Trimix_Enclosure_A3_PrintReview (Autodesk Fusion 360 design; units mm, degrees)
description: Main housing
part number: TMX-A3-P01
description: Single rear cover
part number: TMX-A3-P02
description: Guition display assembly
part number: TMX-A3-C01-V01
part number: TMX-A3-C01-V02
part number: TMX-A3-C01-V03
part number: TMX-A3-C01-V04
description: M3 x 8 button-head screw
part number: TMX-A3-F01
description: M3 heat-set insert, OD4.2 x 5
part number: TMX-A3-F04
description: Electronics carrier
part number: TMX-A3-P03
description: Main electronics PCB
part number: TMX-A3-B01
description: M2 x 7 socket-cap screw
part number: TMX-A3-F03
description: M2 heat-set insert, OD3.2 x 4
part number: TMX-A3-F05
description: Lower display retainer
part number: TMX-A3-P04
description: Upper display retainer
part number: TMX-A3-P05
description: M2 x 5 socket-cap screw
part number: TMX-A3-F02
description: Protected two-cell holder
part number: TMX-A3-C02
description: 18650 cell
part number: TMX-A3-C03-V01
part number: TMX-A3-C03-V02
description: Two-wire battery disconnect pair
part number: TMX-A3-C10-V01
part number: TMX-A3-C10-V02
description: Momentary illuminated 1NO button
part number: TMX-A3-C04-V01
part number: TMX-A3-C04-V02
part number: TMX-A3-C04-V03
description: Printed USB bezel and hidden flange
part number: TMX-A3-P09
description: USB support frame
part number: TMX-A3-P06
description: Printed USB retaining bridge
part number: TMX-A3-P10
description: USB daughterboard
part number: TMX-A3-B02
description: USB-C receptacle
part number: TMX-A3-C05-V01
part number: TMX-A3-C05-V02
part number: TMX-A3-C05-V04
part number: TMX-A3-C05-V03
description: Sampling manifold
part number: TMX-A3-P07
description: Sampling chamber lid
part number: TMX-A3-P08
description: AO2 threaded adapter
part number: TMX-A3-P11
description: Oxygen sensor
part number: TMX-A3-C06
description: AO2 mating cable/connector
part number: TMX-A3-C12
description: Carbon-monoxide module
part number: TMX-A3-C09
description: Thermal-conductivity sensor
part number: TMX-A3-C07
description: Humidity breakout
part number: TMX-A3-C08
description: Gas fitting
part number: TMX-A3-C11-V01
part number: TMX-A3-C11-V02
description: AO2 face seal
part number: TMX-A3-S02
description: Chamber harness closure
part number: TMX-A3-S01
description: Guition 4.3 inch display assembly
part number: TMX-A3-C01
description: Momentary 1NO button assembly
part number: TMX-A3-C04
description: GCT USB4720-03-A connector assembly
part number: TMX-A3-C05
Autodesk Fusion 360 part; units mm, degrees
(part 1 of 7)
ref_plane "WorkPlane1" through (0, 0, 0) normal (0, 0, 1) x (1, 0, 0) in component "01 Shape A housing"
sketch "Flat front Shape A outline" plane through (0, 0, 0) normal (0, 0, 1) x (1, 0, 0) in component "01 Shape A housing"
  line L0 (0, 0) -> (85, 0)
  line L1 (85, 0) -> (85, 180)
  line L2 (85, 180) -> (0, 180)
  line L3 (0, 180) -> (0, 0)
  dimension "d39" = 85
  dimension "d40" = 180
  constraint horizontal L0
  constraint vertical L1
  constraint horizontal L2
  constraint vertical L3
  measures "d39" horizontal distance of L0.start L0.end
  measures "d40" vertical distance of L0.end L1.end
ref_plane "WorkPlane2" through (0, 0, 40.6) normal (0, 0, 1) x (1, 0, 0) in component "01 Shape A housing"
sketch "Gently tapered rear outline" plane through (0, 0, 40.6) normal (0, 0, 1) x (1, 0, 0) in component "01 Shape A housing"
  line L0 (0.25, 0.25) -> (84.75, 0.25)
  line L1 (84.75, 0.25) -> (84.75, 179.75)
  line L2 (84.75, 179.75) -> (0.25, 179.75)
  line L3 (0.25, 179.75) -> (0.25, 0.25)
  dimension "d43" = 0.25
  dimension "d44" = 0.25
  dimension "d45" = 84.5
  dimension "d46" = 179.5
  constraint horizontal L0
  constraint vertical L1
  constraint horizontal L2
  constraint vertical L3
  measures "d43" horizontal distance of origin L0.start
  measures "d44" vertical distance of origin L0.start
  measures "d45" horizontal distance of L0.start L0.end
  measures "d46" vertical distance of L0.end L1.end
loft "Shape A restrained taper" add profiles "Flat front Shape A outline", "Gently tapered rear outline" section 1 contours L0 L1 L2 L3 picked at (28.333333, 120) section 2 contours L0 L1 L2 L3 picked at (28.416667, 60.083333) makes body 1 in component "01 Shape A housing"
fillet "Shape A soft outer corners" radius 8 4 edges at (0.125, 0.125, 20.3) (0.125, 179.875, 20.3) (84.875, 0.125, 20.3) (84.875, 179.875, 20.3) on bodies 1 in component "01 Shape A housing"
ref_plane "WorkPlane3" through (0, 0, 14.5) normal (0, 0, 1) x (1, 0, 0) in component "01 Shape A housing"
sketch "Rear cavity cutting tool sketch" plane through (0, 0, 14.5) normal (0, 0, 1) x (1, 0, 0) in component "01 Shape A housing"
  line L0 (2.4, 2.4) -> (82.6, 2.4)
  line L1 (82.6, 2.4) -> (82.6, 177.6)
  line L2 (82.6, 177.6) -> (2.4, 177.6)
  line L3 (2.4, 177.6) -> (2.4, 2.4)
  dimension "d51" = 2.4
  dimension "d52" = 2.4
  dimension "d53" = 80.2
  dimension "d54" = 175.2
  constraint horizontal L0
  constraint vertical L1
  constraint horizontal L2
  constraint vertical L3
  measures "d51" horizontal distance of origin L0.start
  measures "d52" vertical distance of origin L0.start
  measures "d53" horizontal distance of L0.start L0.end
  measures "d54" vertical distance of L0.end L1.end
extrude "Rear cavity cutting tool" add sketch "Rear cavity cutting tool sketch" along normal blind 43 separate body contours L0 L1 L2 L3 picked at (29.133333, 60.8) makes body 2 in component "01 Shape A housing"
fillet "Inner cavity corner rounds" radius 5.6 4 edges at (2.4, 177.6, 36) (82.6, 177.6, 36) (82.6, 2.4, 36) (2.4, 2.4, 36) on bodies 2 in component "01 Shape A housing"
combine "Rounded rear electronics cavity" operation cut target body 1 tool bodies 2 in component "01 Shape A housing"
ref_plane "WorkPlane4" through (0, 0, 2.4) normal (0, 0, 1) x (1, 0, 0) in component "01 Shape A housing"
sketch "Upper sensor cavity cutting tool sketch" plane through (0, 0, 2.4) normal (0, 0, 1) x (1, 0, 0) in component "01 Shape A housing"
  line L0 (2.4, 128) -> (82.6, 128)
  line L1 (82.6, 128) -> (82.6, 177.6)
  line L2 (82.6, 177.6) -> (2.4, 177.6)
  line L3 (2.4, 177.6) -> (2.4, 128)
  dimension "d61" = 2.4
  dimension "d62" = 128
  dimension "d63" = 80.2
  dimension "d64" = 49.6
  constraint horizontal L0
  constraint vertical L1
  constraint horizontal L2
  constraint vertical L3
  measures "d61" horizontal distance of origin L0.start
  measures "d62" vertical distance of origin L0.start
  measures "d63" horizontal distance of L0.start L0.end
  measures "d64" vertical distance of L0.end L1.end
extrude "Upper sensor cavity cutting tool" add sketch "Upper sensor cavity cutting tool sketch" along normal blind 43 separate body contours L0 L1 L2 L3 picked at (29.133333, 161.066667) makes body 3 in component "01 Shape A housing"
fillet "Upper pod inner top corner rounds" radius 5.6 2 edges at (2.4, 177.6, 23.9) (82.6, 177.6, 23.9) on bodies 3 in component "01 Shape A housing"
combine "Upper sensor pod front clearance" operation cut target body 1 tool bodies 3 in component "01 Shape A housing"
ref_plane "WorkPlane5" through (0, 0, -1) normal (0, 0, 1) x (1, 0, 0) in component "01 Shape A housing"
sketch "Front removable factory display aperture sketch" plane through (0, 0, -1) normal (0, 0, 1) x (1, 0, 0) in component "01 Shape A housing"
  line L0 (7.45, 4.8) -> (77.55, 4.8)
  line L1 (77.55, 4.8) -> (77.55, 122.4)
  line L2 (77.55, 122.4) -> (7.45, 122.4)
  line L3 (7.45, 122.4) -> (7.45, 4.8)
  dimension "d71" = 7.45
  dimension "d72" = 4.8
  dimension "d73" = 70.1
  dimension "d74" = 117.6
  constraint horizontal L0
  constraint vertical L1
  constraint horizontal L2
  constraint vertical L3
  measures "d71" horizontal distance of origin L0.start
  measures "d72" vertical distance of origin L0.start
  measures "d73" horizontal distance of L0.start L0.end
  measures "d74" vertical distance of L0.end L1.end
extrude "Front removable factory display aperture" cut sketch "Front removable factory display aperture sketch" along normal blind 16 contours L0 L1 L2 L3 picked at (30.816667, 83.2) bodies 1 in component "01 Shape A housing"
fillet "Display aperture corner rounds" radius 2.4 4 edges at (77.55, 4.8, 7.25) (7.45, 4.8, 7.25) (7.45, 122.4, 7.25) (77.55, 122.4, 7.25) on bodies 1 in component "01 Shape A housing"
ref_plane "WorkPlane6" through (-1, 0, 0) normal (1, 0, 0) x (0, 1, 0) in component "01 Shape A housing"
sketch "Opposed upper gas fitting clearances sketch" plane through (-1, 0, 0) normal (1, 0, 0) x (0, 0, -1) in component "01 Shape A housing"
  circle A0 centre (-22, 162.5) radius 4.5
  dimension "d82" = 162.5
  dimension "d83" = 4.5
  measures "d82" vertical distance of origin A0.centre
  measures "d83" radius of A0
extrude "Opposed upper gas fitting clearances" cut sketch "Opposed upper gas fitting clearances sketch" along normal blind 87 contours A0 picked at (-22.333781, 163.962392) bodies 1 in component "01 Shape A housing"
ref_plane "WorkPlane7" through (81.6, 0, 0) normal (1, 0, 0) x (0, 1, 0) in component "01 Shape A housing"
sketch "Left-side power button opening sketch" plane through (81.6, 0, 0) normal (1, 0, 0) x (0, 0, -1) in component "01 Shape A housing"
  circle A0 centre (-31, 113) radius 6
  dimension "d89" = 113
  dimension "d90" = 6
  measures "d89" vertical distance of origin A0.centre
  measures "d90" radius of A0
extrude "Left-side power button opening" cut sketch "Left-side power button opening sketch" along normal blind 4.4 contours A0 picked at (-29.46738, 110.75206) bodies 1 in component "01 Shape A housing"
ref_plane "WorkPlane1" through (0, 0, 40.8) normal (0, 0, 1) x (1, 0, 0) in component "02 Single rear cover"
sketch "Single rear cover sketch" plane through (0, 0, 40.8) normal (0, 0, 1) x (1, 0, 0) in component "02 Single rear cover"
  line L0 (0.25, 0.25) -> (84.75, 0.25)
  line L1 (84.75, 0.25) -> (84.75, 179.75)
  line L2 (84.75, 179.75) -> (0.25, 179.75)
  line L3 (0.25, 179.75) -> (0.25, 0.25)
  dimension "d95" = 0.25
  dimension "d96" = 0.25
  dimension "d97" = 84.5
  dimension "d98" = 179.5
  constraint horizontal L0
  constraint vertical L1
  constraint horizontal L2
  constraint vertical L3
  measures "d95" horizontal distance of origin L0.start
  measures "d96" vertical distance of origin L0.start
  measures "d97" horizontal distance of L0.start L0.end
  measures "d98" vertical distance of L0.end L1.end
extrude "Single rear cover" add sketch "Single rear cover sketch" along normal blind 2.2 separate body contours L0 L1 L2 L3 picked at (28.416667, 60.083333) makes body 4 in component "02 Single rear cover"
fillet "Soft rear cover corners" radius 8 4 edges at (0.25, 179.75, 41.9) (84.75, 179.75, 41.9) (84.75, 0.25, 41.9) (0.25, 0.25, 41.9) on bodies 4 in component "02 Single rear cover"
fillet "Soft rear edge roll" radius 0.8 8 edges at (2.593146, 2.593146, 43) (0.25, 90, 43) (42.5, 0.25, 43) (82.406854, 2.593146, 43) (84.75, 90, 43) (82.406854, 177.406854, 43) (42.5, 179.75, 43) (2.593146, 177.406854, 43) on bodies 4 in component "02 Single rear cover"
ref_plane "WorkPlane1" through (0, 0, 0.4) normal (0, 0, 1) x (1, 0, 0) in component "03 Guition factory casing — measured envelope"
sketch "Retained factory frame sketch" plane through (0, 0, 0.4) normal (0, 0, 1) x (1, 0, 0) in component "03 Guition factory casing — measured envelope"
  line L0 (7.85, 5.2) -> (77.15, 5.2)
  line L1 (77.15, 5.2) -> (77.15, 122)
  line L2 (77.15, 122) -> (7.85, 122)
  line L3 (7.85, 122) -> (7.85, 5.2)
  dimension "d107" = 7.85
  dimension "d108" = 5.2
  dimension "d109" = 69.3
  dimension "d110" = 116.8
  constraint horizontal L0
  constraint vertical L1
  constraint horizontal L2
  constraint vertical L3
  measures "d107" horizontal distance of origin L0.start
  measures "d108" vertical distance of origin L0.start
  measures "d109" horizontal distance of L0.start L0.end
  measures "d110" vertical distance of L0.end L1.end
extrude "Retained factory frame" add sketch "Retained factory frame sketch" along normal blind 13.7 separate body contours L0 L1 L2 L3 picked at (30.95, 83.066667) makes body 5 in component "03 Guition factory casing — measured envelope"
fillet "Factory corner reference" radius 2 4 edges at (7.85, 122, 7.25) (77.15, 122, 7.25) (77.15, 5.2, 7.25) (7.85, 5.2, 7.25) on bodies 5 in component "03 Guition factory casing — measured envelope"
ref_plane "WorkPlane2" through (0, 0, 3.4) normal (0, 0, 1) x (1, 0, 0) in component "03 Guition factory casing — measured envelope"
sketch "Factory open rear sketch" plane through (0, 0, 3.4) normal (0, 0, 1) x (1, 0, 0) in component "03 Guition factory casing — measured envelope"
  line L0 (9.8, 9.6) -> (75.2, 9.6)
  line L1 (75.2, 9.6) -> (75.2, 117.6)
  line L2 (75.2, 117.6) -> (9.8, 117.6)
  line L3 (9.8, 117.6) -> (9.8, 9.6)
  dimension "d117" = 9.8
  dimension "d118" = 9.6
  dimension "d119" = 65.4
  dimension "d120" = 108
  constraint horizontal L0
  constraint vertical L1
  constraint horizontal L2
  constraint vertical L3
  measures "d117" horizontal distance of origin L0.start
  measures "d118" vertical distance of origin L0.start
  measures "d119" horizontal distance of L0.start L0.end
  measures "d120" vertical distance of L0.end L1.end
extrude "Factory open rear" cut sketch "Factory open rear sketch" along normal blind 12 contours L0 L1 L2 L3 picked at (31.6, 81.6) bodies 5 in component "03 Guition factory casing — measured envelope"
ref_plane "WorkPlane3" through (0, 0, 0.3) normal (0, 0, 1) x (1, 0, 0) in component "03 Guition factory casing — measured envelope"
sketch "Factory glass recess sketch" plane through (0, 0, 0.3) normal (0, 0, 1) x (1, 0, 0) in component "03 Guition factory casing — measured envelope"
  line L0 (9.1, 6.4) -> (75.9, 6.4)
  line L1 (75.9, 6.4) -> (75.9, 120.8)
  line L2 (75.9, 120.8) -> (9.1, 120.8)
  line L3 (9.1, 120.8) -> (9.1, 6.4)
  dimension "d125" = 9.1
  dimension "d126" = 6.4
  dimension "d127" = 66.8
  dimension "d128" = 114.4
  constraint horizontal L0
  constraint vertical L1
  constraint horizontal L2
  constraint vertical L3
  measures "d125" horizontal distance of origin L0.start
  measures "d126" vertical distance of origin L0.start
  measures "d127" horizontal distance of L0.start L0.end
  measures "d128" vertical distance of L0.end L1.end
extrude "Factory glass recess" cut sketch "Factory glass recess sketch" along normal blind 1.3 contours L0 L1 L2 L3 picked at (31.366667, 82.666667) bodies 5 in component "03 Guition factory casing — measured envelope"
ref_plane "WorkPlane1" through (0, 0, 0.4) normal (0, 0, 1) x (1, 0, 0) in component "04 Guition front glass — drawing reference"
sketch "Factory glass black border sketch" plane through (0, 0, 0.4) normal (0, 0, 1) x (1, 0, 0) in component "04 Guition front glass — drawing reference"
  line L0 (9.1, 6.4) -> (75.9, 6.4)
  line L1 (75.9, 6.4) -> (75.9, 120.8)
  line L2 (75.9, 120.8) -> (9.1, 120.8)
  line L3 (9.1, 120.8) -> (9.1, 6.4)
  dimension "d133" = 9.1
  dimension "d134" = 6.4
  dimension "d135" = 66.8
  dimension "d136" = 114.4
  constraint horizontal L0
  constraint vertical L1
  constraint horizontal L2
  constraint vertical L3
  measures "d133" horizontal distance of origin L0.start
  measures "d134" vertical distance of origin L0.start
  measures "d135" horizontal distance of L0.start L0.end
  measures "d136" vertical distance of L0.end L1.end
extrude "Factory glass black border" add sketch "Factory glass black border sketch" along normal blind 1.2 separate body contours L0 L1 L2 L3 picked at (31.366667, 82.666667) makes body 6 in component "04 Guition front glass — drawing reference"
ref_plane "WorkPlane2" through (0, 0, 0.3) normal (0, 0, 1) x (1, 0, 0) in component "04 Guition front glass — drawing reference"
sketch "Active face recess sketch" plane through (0, 0, 0.3) normal (0, 0, 1) x (1, 0, 0) in component "04 Guition front glass — drawing reference"
  line L0 (14.42, 16.8) -> (70.58, 16.8)
  line L1 (70.58, 16.8) -> (70.58, 110.4)
  line L2 (70.58, 110.4) -> (14.42, 110.4)
  line L3 (14.42, 110.4) -> (14.42, 16.8)
  dimension "d141" = 14.42
  dimension "d142" = 16.8
  dimension "d143" = 56.16
  dimension "d144" = 93.6
  constraint horizontal L0
  constraint vertical L1
  constraint horizontal L2
  constraint vertical L3
  measures "d141" horizontal distance of origin L0.start
  measures "d142" vertical distance of origin L0.start
  measures "d143" horizontal distance of L0.start L0.end
  measures "d144" vertical distance of L0.end L1.end
extrude "Active face recess" cut sketch "Active face recess sketch" along normal blind 0.2 contours L0 L1 L2 L3 picked at (33.14, 48) bodies 6 in component "04 Guition front glass — drawing reference"
ref_plane "WorkPlane1" through (0, 0, 0.4) normal (0, 0, 1) x (1, 0, 0) in component "05 Active 4.3 inch screen"
sketch "Active480x800 screen sketch" plane through (0, 0, 0.4) normal (0, 0, 1) x (1, 0, 0) in component "05 Active 4.3 inch screen"
  line L0 (14.42, 16.8) -> (70.58, 16.8)
  line L1 (70.58, 16.8) -> (70.58, 110.4)
  line L2 (70.58, 110.4) -> (14.42, 110.4)
  line L3 (14.42, 110.4) -> (14.42, 16.8)
  dimension "d149" = 14.42
  dimension "d150" = 16.8
  dimension "d151" = 56.16
  dimension "d152" = 93.6
  constraint horizontal L0
  constraint vertical L1
  constraint horizontal L2
  constraint vertical L3
  measures "d149" horizontal distance of origin L0.start
  measures "d150" vertical distance of origin L0.start
  measures "d151" horizontal distance of L0.start L0.end
  measures "d152" vertical distance of L0.end L1.end
extrude "Active480x800 screen" add sketch "Active480x800 screen sketch" along normal blind 0.1 separate body contours L0 L1 L2 L3 picked at (33.14, 48) makes body 7 in component "05 Active 4.3 inch screen"
ref_plane "WorkPlane1" through (0, 0, 8) normal (0, 0, 1) x (1, 0, 0) in component "06 Guition PCB and connectors — illustrative detail"
sketch "Guition PCB outline sketch" plane through (0, 0, 8) normal (0, 0, 1) x (1, 0, 0) in component "06 Guition PCB and connectors — illustrative detail"
  line L0 (9.97, 9.6) -> (75.03, 9.6)
  line L1 (75.03, 9.6) -> (75.03, 117.6)
  line L2 (75.03, 117.6) -> (9.97, 117.6)
  line L3 (9.97, 117.6) -> (9.97, 9.6)
  dimension "d157" = 9.97
  dimension "d158" = 9.6
  dimension "d159" = 65.06
  dimension "d160" = 108
  constraint horizontal L0
  constraint vertical L1
  constraint horizontal L2
  constraint vertical L3
  measures "d157" horizontal distance of origin L0.start
  measures "d158" vertical distance of origin L0.start
  measures "d159" horizontal distance of L0.start L0.end
  measures "d160" vertical distance of L0.end L1.end
extrude "Guition PCB outline" add sketch "Guition PCB outline sketch" along normal blind 1.6 separate body contours L0 L1 L2 L3 picked at (31.656667, 81.6) makes body 8 in component "06 Guition PCB and connectors — illustrative detail"
ref_plane "WorkPlane2" through (0, 0, 7.9) normal (0, 0, 1) x (1, 0, 0) in component "06 Guition PCB and connectors — illustrative detail"
sketch "Factory mounting-hole reference sketch" plane through (0, 0, 7.9) normal (0, 0, 1) x (1, 0, 0) in component "06 Guition PCB and connectors — illustrative detail"
  circle A0 centre (12.5, 12.3) radius 2.5
  dimension "d165" = 12.5
  dimension "d166" = 12.3
  dimension "d167" = 2.5
  measures "d165" horizontal distance of origin A0.centre
  measures "d166" vertical distance of origin A0.centre
  measures "d167" radius of A0
extrude "Factory mounting-hole reference" cut sketch "Factory mounting-hole reference sketch" along normal blind 1.8 contours A0 picked at (11.518255, 11.733189) bodies 8 in component "06 Guition PCB and connectors — illustrative detail"
ref_plane "WorkPlane3" through (0, 0, 7.9) normal (0, 0, 1) x (1, 0, 0) in component "06 Guition PCB and connectors — illustrative detail"
sketch "Factory mounting-hole reference sketch (1)" plane through (0, 0, 7.9) normal (0, 0, 1) x (1, 0, 0) in component "06 Guition PCB and connectors — illustrative detail"
  circle A0 centre (12.5, 114.9) radius 2.5
  dimension "d172" = 12.5
  dimension "d173" = 114.9
  dimension "d174" = 2.5
  measures "d172" horizontal distance of origin A0.centre
  measures "d173" vertical distance of origin A0.centre
  measures "d174" radius of A0
extrude "Factory mounting-hole reference (1)" cut sketch "Factory mounting-hole reference sketch (1)" along normal blind 1.8 contours A0 picked at (13.287535, 115.621688) bodies 8 in component "06 Guition PCB and connectors — illustrative detail"
ref_plane "WorkPlane4" through (0, 0, 7.9) normal (0, 0, 1) x (1, 0, 0) in component "06 Guition PCB and connectors — illustrative detail"
sketch "Factory mounting-hole reference sketch (2)" plane through (0, 0, 7.9) normal (0, 0, 1) x (1, 0, 0) in component "06 Guition PCB and connectors — illustrative detail"
  circle A0 centre (72.5, 12.3) radius 2.5
  dimension "d179" = 72.5
  dimension "d180" = 12.3
  dimension "d181" = 2.5
  measures "d179" horizontal distance of origin A0.centre
  measures "d180" vertical distance of origin A0.centre
  measures "d181" radius of A0
extrude "Factory mounting-hole reference (2)" cut sketch "Factory mounting-hole reference sketch (2)" along normal blind 1.8 contours A0 picked at (72.060056, 13.42096) bodies 8 in component "06 Guition PCB and connectors — illustrative detail"
ref_plane "WorkPlane5" through (0, 0, 7.9) normal (0, 0, 1) x (1, 0, 0) in component "06 Guition PCB and connectors — illustrative detail"
sketch "Factory mounting-hole reference sketch (3)" plane through (0, 0, 7.9) normal (0, 0, 1) x (1, 0, 0) in component "06 Guition PCB and connectors — illustrative detail"
  circle A0 centre (72.5, 114.9) radius 2.5
  dimension "d186" = 72.5
  dimension "d187" = 114.9
  dimension "d188" = 2.5
  measures "d186" horizontal distance of origin A0.centre
  measures "d187" vertical distance of origin A0.centre
  measures "d188" radius of A0
extrude "Factory mounting-hole reference (3)" cut sketch "Factory mounting-hole reference sketch (3)" along normal blind 1.8 contours A0 picked at (74.260267, 114.705637) bodies 8 in component "06 Guition PCB and connectors — illustrative detail"
ref_plane "WorkPlane6" through (0, 0, 9.6) normal (0, 0, 1) x (1, 0, 0) in component "06 Guition PCB and connectors — illustrative detail"
sketch "ESP32-P4 visual reference sketch" plane through (0, 0, 9.6) normal (0, 0, 1) x (1, 0, 0) in component "06 Guition PCB and connectors — illustrative detail"
  line L0 (20, 76.1) -> (36, 76.1)
  line L1 (36, 76.1) -> (36, 92.1)
  line L2 (36, 92.1) -> (20, 92.1)
  line L3 (20, 92.1) -> (20, 76.1)
  dimension "d193" = 20
  dimension "d194" = 76.1
  dimension "d195" = 16
  dimension "d196" = 16
  constraint horizontal L0
  constraint vertical L1
  constraint horizontal L2
  constraint vertical L3
  measures "d193" horizontal distance of origin L0.start
  measures "d194" vertical distance of origin L0.start
  measures "d195" horizontal distance of L0.start L0.end
  measures "d196" vertical distance of L0.end L1.end
extrude "ESP32-P4 visual reference" add sketch "ESP32-P4 visual reference sketch" along normal blind 3 separate body contours L0 L1 L2 L3 picked at (25.333333, 86.766667) makes body 9 in component "06 Guition PCB and connectors — illustrative detail"
ref_plane "WorkPlane7" through (0, 0, 9.6) normal (0, 0, 1) x (1, 0, 0) in component "06 Guition PCB and connectors — illustrative detail"
sketch "ESP32-C6 visual reference sketch" plane through (0, 0, 9.6) normal (0, 0, 1) x (1, 0, 0) in component "06 Guition PCB and connectors — illustrative detail"
  line L0 (52, 91.1) -> (66, 91.1)
  line L1 (66, 91.1) -> (66, 110.1)
  line L2 (66, 110.1) -> (52, 110.1)
  line L3 (52, 110.1) -> (52, 91.1)
  dimension "d201" = 52
  dimension "d202" = 91.1
  dimension "d203" = 14
  dimension "d204" = 19
  constraint horizontal L0
  constraint vertical L1
  constraint horizontal L2
  constraint vertical L3
  measures "d201" horizontal distance of origin L0.start
  measures "d202" vertical distance of origin L0.start
  measures "d203" horizontal distance of L0.start L0.end
  measures "d204" vertical distance of L0.end L1.end
extrude "ESP32-C6 visual reference" add sketch "ESP32-C6 visual reference sketch" along normal blind 2.8 separate body contours L0 L1 L2 L3 picked at (56.666667, 103.766667) makes body 10 in component "06 Guition PCB and connectors — illustrative detail"
ref_plane "WorkPlane8" through (0, 0, 9.6) normal (0, 0, 1) x (1, 0, 0) in component "06 Guition PCB and connectors — illustrative detail"
sketch "Memory visual reference sketch" plane through (0, 0, 9.6) normal (0, 0, 1) x (1, 0, 0) in component "06 Guition PCB and connectors — illustrative detail"
  line L0 (39, 80.1) -> (46, 80.1)
  line L1 (46, 80.1) -> (46, 89.1)
  line L2 (46, 89.1) -> (39, 89.1)
  line L3 (39, 89.1) -> (39, 80.1)
  dimension "d209" = 39
  dimension "d210" = 80.1
  dimension "d211" = 7
  dimension "d212" = 9
  constraint horizontal L0
  constraint vertical L1
  constraint horizontal L2
  constraint vertical L3
  measures "d209" horizontal distance of origin L0.start
  measures "d210" vertical distance of origin L0.start
  measures "d211" horizontal distance of L0.start L0.end
  measures "d212" vertical distance of L0.end L1.end
extrude "Memory visual reference" add sketch "Memory visual reference sketch" along normal blind 1.2 separate body contours L0 L1 L2 L3 picked at (41.333333, 83.1) makes body 11 in component "06 Guition PCB and connectors — illustrative detail"
ref_plane "WorkPlane9" through (0, 0, 9.6) normal (0, 0, 1) x (1, 0, 0) in component "06 Guition PCB and connectors — illustrative detail"
sketch "Power inductor visual reference sketch" plane through (0, 0, 9.6) normal (0, 0, 1) x (1, 0, 0) in component "06 Guition PCB and connectors — illustrative detail"
  line L0 (19, 19.1) -> (25, 19.1)
  line L1 (25, 19.1) -> (25, 25.1)
  line L2 (25, 25.1) -> (19, 25.1)
  line L3 (19, 25.1) -> (19, 19.1)
  dimension "d217" = 19
  dimension "d218" = 19.1
  dimension "d219" = 6
  dimension "d220" = 6
  constraint horizontal L0
  constraint vertical L1
  constraint horizontal L2
  constraint vertical L3
  measures "d217" horizontal distance of origin L0.start
  measures "d218" vertical distance of origin L0.start
  measures "d219" horizontal distance of L0.start L0.end
  measures "d220" vertical distance of L0.end L1.end
extrude "Power inductor visual reference" add sketch "Power inductor visual reference sketch" along normal blind 3.4 separate body contours L0 L1 L2 L3 picked at (21, 23.1) makes body 12 in component "06 Guition PCB and connectors — illustrative detail"
ref_plane "WorkPlane10" through (0, 0, 9.6) normal (0, 0, 1) x (1, 0, 0) in component "06 Guition PCB and connectors — illustrative detail"
sketch "Power IC visual reference sketch" plane through (0, 0, 9.6) normal (0, 0, 1) x (1, 0, 0) in component "06 Guition PCB and connectors — illustrative detail"
  line L0 (29, 24.1) -> (34, 24.1)
  line L1 (34, 24.1) -> (34, 29.1)
  line L2 (34, 29.1) -> (29, 29.1)
  line L3 (29, 29.1) -> (29, 24.1)
  dimension "d225" = 29
  dimension "d226" = 24.1
  dimension "d227" = 5
  dimension "d228" = 5
  constraint horizontal L0
  constraint vertical L1
  constraint horizontal L2
  constraint vertical L3
  measures "d225" horizontal distance of origin L0.start
  measures "d226" vertical distance of origin L0.start
  measures "d227" horizontal distance of L0.start L0.end
  measures "d228" vertical distance of L0.end L1.end
extrude "Power IC visual reference" add sketch "Power IC visual reference sketch" along normal blind 1.5 separate body contours L0 L1 L2 L3 picked at (30.666667, 27.433333) makes body 13 in component "06 Guition PCB and connectors — illustrative detail"
ref_plane "WorkPlane11" through (0, 0, 9.6) normal (0, 0, 1) x (1, 0, 0) in component "06 Guition PCB and connectors — illustrative detail"
sketch "Factory USB visual reference sketch" plane through (0, 0, 9.6) normal (0, 0, 1) x (1, 0, 0) in component "06 Guition PCB and connectors — illustrative detail"
  line L0 (35, 10.1) -> (44, 10.1)
  line L1 (44, 10.1) -> (44, 17.1)
  line L2 (44, 17.1) -> (35, 17.1)
  line L3 (35, 17.1) -> (35, 10.1)
  dimension "d233" = 35
  dimension "d234" = 10.1
  dimension "d235" = 9
  dimension "d236" = 7
  constraint horizontal L0
  constraint vertical L1
  constraint horizontal L2
  constraint vertical L3
  measures "d233" horizontal distance of origin L0.start
  measures "d234" vertical distance of origin L0.start
  measures "d235" horizontal distance of L0.start L0.end
  measures "d236" vertical distance of L0.end L1.end
extrude "Factory USB visual reference" add sketch "Factory USB visual reference sketch" along normal blind 3.8 separate body contours L0 L1 L2 L3 picked at (38, 14.766667) makes body 14 in component "06 Guition PCB and connectors — illustrative detail"
ref_plane "WorkPlane12" through (0, 0, 9.6) normal (0, 0, 1) x (1, 0, 0) in component "06 Guition PCB and connectors — illustrative detail"
sketch "FPC latch visual reference sketch" plane through (0, 0, 9.6) normal (0, 0, 1) x (1, 0, 0) in component "06 Guition PCB and connectors — illustrative detail"
  line L0 (28, 63.1) -> (56, 63.1)
  line L1 (56, 63.1) -> (56, 67.1)
  line L2 (56, 67.1) -> (28, 67.1)
  line L3 (28, 67.1) -> (28, 63.1)
  dimension "d241" = 28
  dimension "d242" = 63.1
  dimension "d243" = 28
  dimension "d244" = 4
  constraint horizontal L0
  constraint vertical L1
  constraint horizontal L2
  constraint vertical L3
  measures "d241" horizontal distance of origin L0.start
  measures "d242" vertical distance of origin L0.start
  measures "d243" horizontal distance of L0.start L0.end
  measures "d244" vertical distance of L0.end L1.end
extrude "FPC latch visual reference" add sketch "FPC latch visual reference sketch" along normal blind 1.8 separate body contours L0 L1 L2 L3 picked at (37.333333, 65.766667) makes body 15 in component "06 Guition PCB and connectors — illustrative detail"
ref_plane "WorkPlane13" through (0, 0, 9.6) normal (0, 0, 1) x (1, 0, 0) in component "06 Guition PCB and connectors — illustrative detail"
sketch "Expansion header visual reference sketch" plane through (0, 0, 9.6) normal (0, 0, 1) x (1, 0, 0) in component "06 Guition PCB and connectors — illustrative detail"
  line L0 (57, 35.1) -> (62, 35.1)
  line L1 (62, 35.1) -> (62, 68.1)
  line L2 (62, 68.1) -> (57, 68.1)
  line L3 (57, 68.1) -> (57, 35.1)
  dimension "d249" = 57
  dimension "d250" = 35.1
  dimension "d251" = 5
  dimension "d252" = 33
  constraint horizontal L0
  constraint vertical L1
  constraint horizontal L2
  constraint vertical L3
  measures "d249" horizontal distance of origin L0.start
  measures "d250" vertical distance of origin L0.start
  measures "d251" horizontal distance of L0.start L0.end
  measures "d252" vertical distance of L0.end L1.end
extrude "Expansion header visual reference" add sketch "Expansion header visual reference sketch" along normal blind 4 separate body contours L0 L1 L2 L3 picked at (58.666667, 57.1) makes body 16 in component "06 Guition PCB and connectors — illustrative detail"
ref_plane "WorkPlane8" through (0, 0, 30) normal (0, 0, 1) x (1, 0, 0) in component "01 Shape A housing"
sketch "Rear boss end-wall web sketch" plane through (0, 0, 30) normal (0, 0, 1) x (1, 0, 0) in component "01 Shape A housing"
  line L0 (4.3, 2.3) -> (11.7, 2.3)
  line L1 (11.7, 2.3) -> (11.7, 11.5)
  line L2 (11.7, 11.5) -> (4.3, 11.5)
  line L3 (4.3, 11.5) -> (4.3, 2.3)
  dimension "d257" = 4.3
  dimension "d258" = 2.3
  dimension "d259" = 7.4
  dimension "d260" = 9.2
  constraint horizontal L0
  constraint vertical L1
  constraint horizontal L2
  constraint vertical L3
  measures "d257" horizontal distance of origin L0.start
  measures "d258" vertical distance of origin L0.start
  measures "d259" horizontal distance of L0.start L0.end
  measures "d260" vertical distance of L0.end L1.end
extrude "Rear boss end-wall web" add sketch "Rear boss end-wall web sketch" along normal blind 9 contours L0 L1 L2 L3 picked at (9.233333, 5.366667) bodies 1 in component "01 Shape A housing"
ref_plane "WorkPlane9" through (0, 0, 30) normal (0, 0, 1) x (1, 0, 0) in component "01 Shape A housing"
sketch "Rear M3 boss sketch" plane through (0, 0, 30) normal (0, 0, 1) x (1, 0, 0) in component "01 Shape A housing"
  circle A0 centre (8, 8) radius 4.2
  dimension "d265" = 8
  dimension "d266" = 8
  dimension "d267" = 4.2
  measures "d265" horizontal distance of origin A0.centre
  measures "d266" vertical distance of origin A0.centre
  measures "d267" radius of A0
extrude "Rear M3 boss" add sketch "Rear M3 boss sketch" along normal blind 9 contours A0 picked at (9.026273, 7.047758) bodies 1 in component "01 Shape A housing"
ref_plane "WorkPlane10" through (0, 0, 34) normal (0, 0, 1) x (1, 0, 0) in component "01 Shape A housing"
sketch "M3 insert pilot sketch" plane through (0, 0, 34) normal (0, 0, 1) x (1, 0, 0) in component "01 Shape A housing"
  circle A0 centre (8, 8) radius 2.15
  dimension "d272" = 8
  dimension "d273" = 8
  dimension "d274" = 2.15
  measures "d272" horizontal distance of origin A0.centre
  measures "d273" vertical distance of origin A0.centre
  measures "d274" radius of A0
extrude "M3 insert pilot" cut sketch "M3 insert pilot sketch" along normal blind 5.1 contours A0 picked at (7.641667, 7.379348) bodies 1 in component "01 Shape A housing"
ref_plane "WorkPlane2" through (0, 0, 39.2) normal (0, 0, 1) x (1, 0, 0) in component "02 Single rear cover"
sketch "Reinforced rear screw seat sketch" plane through (0, 0, 39.2) normal (0, 0, 1) x (1, 0, 0) in component "02 Single rear cover"
  circle A0 centre (8, 8) radius 4.8
  dimension "d279" = 8
  dimension "d280" = 8
  dimension "d281" = 4.8
  measures "d279" horizontal distance of origin A0.centre
  measures "d280" vertical distance of origin A0.centre
  measures "d281" radius of A0
extrude "Reinforced rear screw seat" add sketch "Reinforced rear screw seat sketch" along normal blind 2.15 contours A0 picked at (5.638882, 8.904099) bodies 4 in component "02 Single rear cover"
ref_plane "WorkPlane3" through (0, 0, 39.1) normal (0, 0, 1) x (1, 0, 0) in component "02 Single rear cover"
sketch "M3 screw clearance sketch" plane through (0, 0, 39.1) normal (0, 0, 1) x (1, 0, 0) in component "02 Single rear cover"
  circle A0 centre (8, 8) radius 1.65
  dimension "d286" = 8
  dimension "d287" = 8
  dimension "d288" = 1.65
  measures "d286" horizontal distance of origin A0.centre
  measures "d287" vertical distance of origin A0.centre
  measures "d288" radius of A0
extrude "M3 screw clearance" cut sketch "M3 screw clearance sketch" along normal blind 4.1 contours A0 picked at (8.409322, 8.456068) bodies 4 in component "02 Single rear cover"
ref_plane "WorkPlane4" through (0, 0, 41.35) normal (0, 0, 1) x (1, 0, 0) in component "02 Single rear cover"
sketch "Flush M3 head recess sketch" plane through (0, 0, 41.35) normal (0, 0, 1) x (1, 0, 0) in component "02 Single rear cover"
  circle A0 centre (8, 8) radius 3
  dimension "d293" = 8
  dimension "d294" = 8
  dimension "d295" = 3
  measures "d293" horizontal distance of origin A0.centre
  measures "d294" vertical distance of origin A0.centre
  measures "d295" radius of A0
extrude "Flush M3 head recess" cut sketch "Flush M3 head recess sketch" along normal blind 1.8 contours A0 picked at (6.936439, 8.848162) bodies 4 in component "02 Single rear cover"
ref_plane "WorkPlane11" through (0, 0, 39.1) normal (0, 0, 1) x (1, 0, 0) in component "01 Shape A housing"
sketch "Cover bearing-pad clearance sketch" plane through (0, 0, 39.1) normal (0, 0, 1) x (1, 0, 0) in component "01 Shape A housing"
  circle A0 centre (8, 8) radius 4.9
  dimension "d300" = 8
  dimension "d301" = 8
  dimension "d302" = 4.9
  measures "d300" horizontal distance of origin A0.centre
  measures "d301" vertical distance of origin A0.centre
  measures "d302" radius of A0
ref_plane "WorkPlane12" through (0, 0, 30) normal (0, 0, 1) x (1, 0, 0) in component "01 Shape A housing"
sketch "Rear boss end-wall web sketch (1)" plane through (0, 0, 30) normal (0, 0, 1) x (1, 0, 0) in component "01 Shape A housing"
  line L0 (73.3, 2.3) -> (80.7, 2.3)
  line L1 (80.7, 2.3) -> (80.7, 11.5)
  line L2 (80.7, 11.5) -> (73.3, 11.5)
  line L3 (73.3, 11.5) -> (73.3, 2.3)
  dimension "d307" = 73.3
  dimension "d308" = 2.3
  dimension "d309" = 7.4
  dimension "d310" = 9.2
  constraint horizontal L0
  constraint vertical L1
  constraint horizontal L2
  constraint vertical L3
  measures "d307" horizontal distance of origin L0.start
  measures "d308" vertical distance of origin L0.start
  measures "d309" horizontal distance of L0.start L0.end
  measures "d310" vertical distance of L0.end L1.end
extrude "Rear boss end-wall web (1)" add sketch "Rear boss end-wall web sketch (1)" along normal blind 9 contours L0 L1 L2 L3 picked at (75.766667, 8.433333) bodies 1 in component "01 Shape A housing"
ref_plane "WorkPlane13" through (0, 0, 30) normal (0, 0, 1) x (1, 0, 0) in component "01 Shape A housing"
sketch "Rear M3 boss sketch (1)" plane through (0, 0, 30) normal (0, 0, 1) x (1, 0, 0) in component "01 Shape A housing"
  circle A0 centre (77, 8) radius 4.2
  dimension "d315" = 77
  dimension "d316" = 8
  dimension "d317" = 4.2
  measures "d315" horizontal distance of origin A0.centre
  measures "d316" vertical distance of origin A0.centre
  measures "d317" radius of A0
extrude "Rear M3 boss (1)" add sketch "Rear M3 boss sketch (1)" along normal blind 9 contours A0 picked at (77.493093, 9.181249) bodies 1 in component "01 Shape A housing"
ref_plane "WorkPlane14" through (0, 0, 34) normal (0, 0, 1) x (1, 0, 0) in component "01 Shape A housing"
sketch "M3 insert pilot sketch (1)" plane through (0, 0, 34) normal (0, 0, 1) x (1, 0, 0) in component "01 Shape A housing"
  circle A0 centre (77, 8) radius 2.15
  dimension "d322" = 77
  dimension "d323" = 8
  dimension "d324" = 2.15
  measures "d322" horizontal distance of origin A0.centre
  measures "d323" vertical distance of origin A0.centre
  measures "d324" radius of A0
extrude "M3 insert pilot (1)" cut sketch "M3 insert pilot sketch (1)" along normal blind 5.1 contours A0 picked at (77.553947, 8.560313) bodies 1 in component "01 Shape A housing"
ref_plane "WorkPlane5" through (0, 0, 39.2) normal (0, 0, 1) x (1, 0, 0) in component "02 Single rear cover"
sketch "Reinforced rear screw seat sketch (1)" plane through (0, 0, 39.2) normal (0, 0, 1) x (1, 0, 0) in component "02 Single rear cover"
  circle A0 centre (77, 8) radius 4.8
  dimension "d329" = 77
  dimension "d330" = 8
  dimension "d331" = 4.8
  measures "d329" horizontal distance of origin A0.centre
  measures "d330" vertical distance of origin A0.centre
  measures "d331" radius of A0
extrude "Reinforced rear screw seat (1)" add sketch "Reinforced rear screw seat sketch (1)" along normal blind 2.15 contours A0 picked at (73.585567, 8.991578) bodies 4 in component "02 Single rear cover"
ref_plane "WorkPlane6" through (0, 0, 39.1) normal (0, 0, 1) x (1, 0, 0) in component "02 Single rear cover"
sketch "M3 screw clearance sketch (1)" plane through (0, 0, 39.1) normal (0, 0, 1) x (1, 0, 0) in component "02 Single rear cover"
  circle A0 centre (77, 8) radius 1.65
  dimension "d336" = 77
  dimension "d337" = 8
  dimension "d338" = 1.65
  measures "d336" horizontal distance of origin A0.centre
  measures "d337" vertical distance of origin A0.centre
  measures "d338" radius of A0
extrude "M3 screw clearance (1)" cut sketch "M3 screw clearance sketch (1)" along normal blind 4.1 contours A0 picked at (76.412308, 7.569993) bodies 4 in component "02 Single rear cover"
ref_plane "WorkPlane7" through (0, 0, 41.35) normal (0, 0, 1) x (1, 0, 0) in component "02 Single rear cover"
sketch "Flush M3 head recess sketch (1)" plane through (0, 0, 41.35) normal (0, 0, 1) x (1, 0, 0) in component "02 Single rear cover"
  circle A0 centre (77, 8) radius 3
  dimension "d343" = 77
  dimension "d344" = 8
  dimension "d345" = 3
  measures "d343" horizontal distance of origin A0.centre
  measures "d344" vertical distance of origin A0.centre
  measures "d345" radius of A0
extrude "Flush M3 head recess (1)" cut sketch "Flush M3 head recess sketch (1)" along normal blind 1.8 contours A0 picked at (76.255779, 8.53113) bodies 4 in component "02 Single rear cover"
ref_plane "WorkPlane15" through (0, 0, 39.1) normal (0, 0, 1) x (1, 0, 0) in component "01 Shape A housing"
sketch "Cover bearing-pad clearance sketch (1)" plane through (0, 0, 39.1) normal (0, 0, 1) x (1, 0, 0) in component "01 Shape A housing"
  circle A0 centre (77, 8) radius 4.9
  dimension "d350" = 77
  dimension "d351" = 8
  dimension "d352" = 4.9
  measures "d350" horizontal distance of origin A0.centre
  measures "d351" vertical distance of origin A0.centre
  measures "d352" radius of A0
ref_plane "WorkPlane16" through (0, 0, 30) normal (0, 0, 1) x (1, 0, 0) in component "01 Shape A housing"
sketch "Rear boss end-wall web sketch (2)" plane through (0, 0, 30) normal (0, 0, 1) x (1, 0, 0) in component "01 Shape A housing"
  line L0 (4.3, 168.5) -> (11.7, 168.5)
  line L1 (11.7, 168.5) -> (11.7, 177.7)
  line L2 (11.7, 177.7) -> (4.3, 177.7)
  line L3 (4.3, 177.7) -> (4.3, 168.5)
  dimension "d357" = 4.3
  dimension "d358" = 168.5
  dimension "d359" = 7.4
  dimension "d360" = 9.2
  constraint horizontal L0
  constraint vertical L1
  constraint horizontal L2
  constraint vertical L3
  measures "d357" horizontal distance of origin L0.start
  measures "d358" vertical distance of origin L0.start
  measures "d359" horizontal distance of L0.start L0.end
  measures "d360" vertical distance of L0.end L1.end
extrude "Rear boss end-wall web (2)" add sketch "Rear boss end-wall web sketch (2)" along normal blind 9 contours L0 L1 L2 L3 picked at (6.766667, 174.633333) bodies 1 in component "01 Shape A housing"
ref_plane "WorkPlane17" through (0, 0, 30) normal (0, 0, 1) x (1, 0, 0) in component "01 Shape A housing"
sketch "Rear M3 boss sketch (2)" plane through (0, 0, 30) normal (0, 0, 1) x (1, 0, 0) in component "01 Shape A housing"
  circle A0 centre (8, 172) radius 4.2
  dimension "d365" = 8
  dimension "d366" = 172
  dimension "d367" = 4.2
  measures "d365" horizontal distance of origin A0.centre
  measures "d366" vertical distance of origin A0.centre
  measures "d367" radius of A0
extrude "Rear M3 boss (2)" add sketch "Rear M3 boss sketch (2)" along normal blind 9 contours A0 picked at (7.688471, 174.942195) bodies 1 in component "01 Shape A housing"
ref_plane "WorkPlane18" through (0, 0, 34) normal (0, 0, 1) x (1, 0, 0) in component "01 Shape A housing"
sketch "M3 insert pilot sketch (2)" plane through (0, 0, 34) normal (0, 0, 1) x (1, 0, 0) in component "01 Shape A housing"
  circle A0 centre (8, 172) radius 2.15
  dimension "d372" = 8
  dimension "d373" = 172
  dimension "d374" = 2.15
  measures "d372" horizontal distance of origin A0.centre
  measures "d373" vertical distance of origin A0.centre
  measures "d374" radius of A0
extrude "M3 insert pilot (2)" cut sketch "M3 insert pilot sketch (2)" along normal blind 5.1 contours A0 picked at (7.553166, 171.439687) bodies 1 in component "01 Shape A housing"
ref_plane "WorkPlane8" through (0, 0, 39.2) normal (0, 0, 1) x (1, 0, 0) in component "02 Single rear cover"
sketch "Reinforced rear screw seat sketch (2)" plane through (0, 0, 39.2) normal (0, 0, 1) x (1, 0, 0) in component "02 Single rear cover"
  circle A0 centre (8, 172) radius 4.8
  dimension "d380" = 172
  dimension "d381" = 4.8
  measures "d379" distance of origin A0.centre
  measures "d380" vertical distance of origin A0.centre
  measures "d381" radius of A0
extrude "Reinforced rear screw seat (2)" add sketch "Reinforced rear screw seat sketch (2)" along normal blind 2.15 contours A0 picked at (5.846383, 171.305786) bodies 4 in component "02 Single rear cover"
ref_plane "WorkPlane9" through (0, 0, 39.1) normal (0, 0, 1) x (1, 0, 0) in component "02 Single rear cover"
sketch "M3 screw clearance sketch (2)" plane through (0, 0, 39.1) normal (0, 0, 1) x (1, 0, 0) in component "02 Single rear cover"
  circle A0 centre (8, 172) radius 1.65
  dimension "d386" = 8
  dimension "d387" = 172
  dimension "d388" = 1.65
  measures "d386" horizontal distance of origin A0.centre
  measures "d387" vertical distance of origin A0.centre
  measures "d388" radius of A0
extrude "M3 screw clearance (2)" cut sketch "M3 screw clearance sketch (2)" along normal blind 4.1 contours A0 picked at (7.877613, 172.53621) bodies 4 in component "02 Single rear cover"
ref_plane "WorkPlane10" through (0, 0, 41.35) normal (0, 0, 1) x (1, 0, 0) in component "02 Single rear cover"
sketch "Flush M3 head recess sketch (2)" plane through (0, 0, 41.35) normal (0, 0, 1) x (1, 0, 0) in component "02 Single rear cover"
  circle A0 centre (8, 172) radius 3
  dimension "d393" = 8
  dimension "d394" = 172
  dimension "d395" = 3
  measures "d393" horizontal distance of origin A0.centre
  measures "d394" vertical distance of origin A0.centre
  measures "d395" radius of A0
extrude "Flush M3 head recess (2)" cut sketch "Flush M3 head recess sketch (2)" along normal blind 1.8 contours A0 picked at (7.832083, 174.240697) bodies 4 in component "02 Single rear cover"
ref_plane "WorkPlane19" through (0, 0, 39.1) normal (0, 0, 1) x (1, 0, 0) in component "01 Shape A housing"
sketch "Cover bearing-pad clearance sketch (2)" plane through (0, 0, 39.1) normal (0, 0, 1) x (1, 0, 0) in component "01 Shape A housing"
  circle A0 centre (8, 172) radius 4.9
  dimension "d400" = 8
  dimension "d401" = 172
  dimension "d402" = 4.9
  measures "d400" horizontal distance of origin A0.centre
  measures "d401" vertical distance of origin A0.centre
  measures "d402" radius of A0
ref_plane "WorkPlane20" through (0, 0, 30) normal (0, 0, 1) x (1, 0, 0) in component "01 Shape A housing"
sketch "Rear boss end-wall web sketch (3)" plane through (0, 0, 30) normal (0, 0, 1) x (1, 0, 0) in component "01 Shape A housing"
  line L0 (73.3, 169.5) -> (80.7, 169.5)
  line L1 (80.7, 169.5) -> (80.7, 177.7)
  line L2 (80.7, 177.7) -> (73.3, 177.7)
  line L3 (73.3, 177.7) -> (73.3, 169.5)
  dimension "d407" = 73.3
  dimension "d408" = 169.5
  dimension "d409" = 7.4
  dimension "d410" = 8.2
  constraint horizontal L0
  constraint vertical L1
  constraint horizontal L2
  constraint vertical L3
  measures "d407" horizontal distance of origin L0.start
  measures "d408" vertical distance of origin L0.start
  measures "d409" horizontal distance of L0.start L0.end
  measures "d410" vertical distance of L0.end L1.end
extrude "Rear boss end-wall web (3)" add sketch "Rear boss end-wall web sketch (3)" along normal blind 9 contours L0 L1 L2 L3 picked at (75.766667, 172.233333) bodies 1 in component "01 Shape A housing"
ref_plane "WorkPlane21" through (0, 0, 30) normal (0, 0, 1) x (1, 0, 0) in component "01 Shape A housing"
sketch "Rear M3 boss sketch (3)" plane through (0, 0, 30) normal (0, 0, 1) x (1, 0, 0) in component "01 Shape A housing"
  circle A0 centre (77, 172) radius 4.2
  dimension "d415" = 77
  dimension "d416" = 172
  dimension "d417" = 4.2
  measures "d415" horizontal distance of origin A0.centre
  measures "d416" vertical distance of origin A0.centre
  measures "d417" radius of A0
extrude "Rear M3 boss (3)" add sketch "Rear M3 boss sketch (3)" along normal blind 9 contours A0 picked at (77.561356, 172.604998) bodies 1 in component "01 Shape A housing"
ref_plane "WorkPlane22" through (0, 0, 34) normal (0, 0, 1) x (1, 0, 0) in component "01 Shape A housing"
sketch "M3 insert pilot sketch (3)" plane through (0, 0, 34) normal (0, 0, 1) x (1, 0, 0) in component "01 Shape A housing"
  circle A0 centre (77, 172) radius 2.15
  dimension "d422" = 77
  dimension "d423" = 172
  dimension "d424" = 2.15
  measures "d422" horizontal distance of origin A0.centre
  measures "d423" vertical distance of origin A0.centre
  measures "d424" radius of A0
extrude "M3 insert pilot (3)" cut sketch "M3 insert pilot sketch (3)" along normal blind 5.1 contours A0 picked at (76.442807, 172.698698) bodies 1 in component "01 Shape A housing"
ref_plane "WorkPlane11" through (0, 0, 39.2) normal (0, 0, 1) x (1, 0, 0) in component "02 Single rear cover"
sketch "Reinforced rear screw seat sketch (3)" plane through (0, 0, 39.2) normal (0, 0, 1) x (1, 0, 0) in component "02 Single rear cover"
  circle A0 centre (77, 172) radius 4.8
  dimension "d429" = 77
  dimension "d430" = 172
  dimension "d431" = 4.8
  measures "d429" horizontal distance of origin A0.centre
  measures "d430" vertical distance of origin A0.centre
  measures "d431" radius of A0
extrude "Reinforced rear screw seat (3)" add sketch "Reinforced rear screw seat sketch (3)" along normal blind 2.15 contours A0 picked at (74.965951, 171.098688) bodies 4 in component "02 Single rear cover"
ref_plane "WorkPlane12" through (0, 0, 39.1) normal (0, 0, 1) x (1, 0, 0) in component "02 Single rear cover"
sketch "M3 screw clearance sketch (3)" plane through (0, 0, 39.1) normal (0, 0, 1) x (1, 0, 0) in component "02 Single rear cover"
  circle A0 centre (77, 172) radius 1.65
  dimension "d436" = 77
  dimension "d437" = 172
  dimension "d438" = 1.65
  measures "d436" horizontal distance of origin A0.centre
  measures "d437" vertical distance of origin A0.centre
  measures "d438" radius of A0
extrude "M3 screw clearance (3)" cut sketch "M3 screw clearance sketch (3)" along normal blind 4.1 contours A0 picked at (76.412308, 171.569993) bodies 4 in component "02 Single rear cover"
ref_plane "WorkPlane13" through (0, 0, 41.35) normal (0, 0, 1) x (1, 0, 0) in component "02 Single rear cover"